Beilagscheiben_v1 (Autodesk Fusion 360 design; units mm, degrees)
Autodesk Fusion 360 part; units mm, degrees
cylinder "Grundkörper Zylinder2" add diameter 9 height 0.8 placed x (1, 0, 0) y (0, 0, -1) z (0, 1, 0) at (0, 0, 0) makes body 1
cylinder "Grundkörper Zylinder3" cut diameter 4.3 height 1 placed x (1, 0, 0) y (0, 0, -1) z (0, 1, 0) at (0, 0, 0) bodies 1
copy_body "Körper kopieren/einfügen1" bodies 1 makes body 2
copy_body "Körper->Berechn1" bodies 1 removing the originals makes body 3 in component "M4"
scale "Maßstab1" factor 1.25 about (0, 0, 0) bodies 2
copy_body "Körper->Berechn2" bodies 2 removing the originals makes body 4 in component "M5"
copy_body "Körper kopieren/einfügen2" bodies 4 makes body 5
scale "Maßstab2" factor 1.2 about (0, 0, 0) bodies 5
copy_body "Körper->Berechn3" bodies 5 removing the originals makes body 6 in component "M6"
copy_body "Körper kopieren/einfügen4" bodies 3 makes body 7
scale "Maßstab3" factor 2 about (0, 0, 0) bodies 7
move_face "Flächen versetzen1" offset 0.1 1 faces at (4.2786, 1.0667, 0.4281) on bodies 7
move_face "Flächen versetzen2" offset -1 1 faces at (8.9553, 1.0667, 0.8961) on bodies 7
copy_body "Körper kopieren/einfügen5" bodies 7 makes body 8
copy_body "Körper kopieren/einfügen6" bodies 8 makes body 9
copy_body "Körper kopieren/einfügen7" bodies 9 makes body 10
copy_body "Körper kopieren/einfügen8" bodies 10 makes body 11
copy_body "Körper->Berechn4" bodies 7 removing the originals makes body 12 in component "M8"
scale "Maßstab4" factor 1.25 about (0, 0, 0) bodies 8
copy_body "Körper->Berechn5" bodies 8 removing the originals makes body 13 in component "M10"
scale "Maßstab5" factor 1.5 about (0, 0, 0) bodies 9
copy_body "Körper->Berechn6" bodies 9 removing the originals makes body 14 in component "M12"
scale "Maßstab6" factor 1.75 about (0, 0, 0) bodies 10
move_face "Flächen versetzen3" offset -0.15 1 faces at (7.3135, 1.8667, 0.7318) on bodies 10
copy_body "Körper->Berechn7" bodies 10 removing the originals makes body 15 in component "M14"
scale "Maßstab7" factor 2 about (0, 0, 0) bodies 11
move_face "Flächen versetzen4" offset -0.1 1 faces at (8.3583, 2.1333, 0.8364) on bodies 11
move_face "Flächen versetzen5" offset -1 1 faces at (15.9205, 2.1333, 1.5931) on bodies 11
copy_body "Körper->Berechn8" bodies 11 removing the originals makes body 16 in component "M16"
component "M4" placed x (1, 0, 0) y (0, 1, 0) z (0, 0, 1) at (0, 0, 0)
component "M5" placed x (1, 0, 0) y (0, 1, 0) z (0, 0, 1) at (0, 0, 0)
component "M6" placed x (1, 0, 0) y (0, 1, 0) z (0, 0, 1) at (0, 0, 0)
component "M8" placed x (1, 0, 0) y (0, 1, 0) z (0, 0, 1) at (0, 0, 0)
component "M10" placed x (1, 0, 0) y (0, 1, 0) z (0, 0, 1) at (0, 0, 0)
component "M12" placed x (1, 0, 0) y (0, 1, 0) z (0, 0, 1) at (0, 0, 0)
component "M14" placed x (1, 0, 0) y (0, 1, 0) z (0, 0, 1) at (0, 0, 0)
component "M16" placed x (1, 0, 0) y (0, 1, 0) z (0, 0, 1) at (0, 0, 0)
named bodies: "M6", "M8", "M10", "M8 (1)", "M12", "M8 (1) (1)", "M14", "M8 (1) (1) (1)", "M16"
